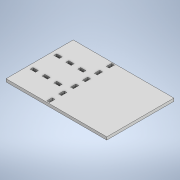
# Autodesk Inventor part: mdf_base_6x6
Saved by Autodesk Inventor 2021.2 (Build 252289000, 289)
## iProperties
Created: 2021-03-24
Part Number: mdf_base_6x6
Material: Generic
Document SubType Name: Modeling
Designer: yxion
Density: 1 g/cm^3
Appearance: Default
Author: yxion
Autodesk Inventor part; units mm, degrees
ref_plane "YZ Plane" through (0, 0, 0) normal (1, 0, 0) x (0, 1, 0)
ref_plane "XZ Plane" through (0, 0, 0) normal (0, 1, 0) x (-1, 0, 0)
ref_plane "XY Plane" through (0, 0, 0) normal (0, 0, 1) x (1, 0, 0)
sketch "Sketch1" plane through (0, 0, 0) normal (0, 1, 0) x (-1, 0, 0)
  line L0 (55.1775, 69.7485) -> (-173.4225, 69.7485)
  line L1 (-173.4225, 69.7485) -> (-173.4225, -82.6515)
  line L2 (-173.4225, -82.6515) -> (55.1775, -82.6515)
  line L3 (55.1775, -82.6515) -> (55.1775, 69.7485)
  point P0 (0, 0)
  dimension "d0" = 152.4
  dimension "d1" = 228.6
  constraints: 8 end point, 2 parallel, 1 horizontal, 1 perpendicular
  measures "d0" distance of L2.end L0.start
  measures "d1" distance of L0.start L0.end
extrude "Extrusion1" add sketch "Sketch1" along normal blind 6.4
sketch "Sketch2" plane through (0, 6.4, 0) normal (0, 1, 0) x (1, 0, 0)
  line L0 (34.6225, 25.9515) -> (41.0225, 25.9515)
  line L1 (41.0225, 25.9515) -> (41.0225, 13.9515)
  line L2 (41.0225, 13.9515) -> (34.6225, 13.9515)
  line L3 (34.6225, 13.9515) -> (34.6225, 25.9515)
  line L4 (34.6225, -1.0485) -> (41.0225, -1.0485)
  line L5 (41.0225, -1.0485) -> (41.0225, -13.0485)
  line L6 (41.0225, -13.0485) -> (34.6225, -13.0485)
  line L7 (34.6225, -13.0485) -> (34.6225, -1.0485)
  line L8 (-55.1775, 82.6515) -> (-55.1775, -69.7485) projected
  line L9 (173.4225, -69.7485) -> (173.4225, 82.6515) construction
  line L10 (173.4225, 82.6515) -> (-55.1775, 82.6515) construction
  line L11 (59.1225, 82.6515) -> (59.1225, -69.7485) construction
  line L12 (-55.1775, -69.7485) -> (173.4225, -69.7485) construction
  line L13 (-55.1775, 6.4515) -> (173.4225, 6.4515) construction
  line L14 (41.0225, -28.0485) -> (41.0225, -40.0485)
  line L15 (34.6225, -40.0485) -> (34.6225, -28.0485)
  line L16 (41.0225, -40.0485) -> (34.6225, -40.0485)
  line L17 (34.6225, -28.0485) -> (41.0225, -28.0485)
  line L18 (41.0225, -55.0485) -> (41.0225, -67.0485)
  line L19 (34.6225, -67.0485) -> (34.6225, -55.0485)
  line L20 (41.0225, -67.0485) -> (34.6225, -67.0485)
  line L21 (34.6225, -55.0485) -> (41.0225, -55.0485)
  line L22 (41.0225, 52.9515) -> (41.0225, 40.9515)
  line L23 (34.6225, 40.9515) -> (34.6225, 52.9515)
  line L24 (34.6225, 52.9515) -> (41.0225, 52.9515)
  line L25 (41.0225, 40.9515) -> (34.6225, 40.9515)
  line L26 (41.0225, 79.9515) -> (41.0225, 67.9515)
  line L27 (34.6225, 67.9515) -> (34.6225, 79.9515)
  line L28 (34.6225, 79.9515) -> (41.0225, 79.9515)
  line L29 (41.0225, 67.9515) -> (34.6225, 67.9515)
  line L30 (7.6225, -17.3485) -> (19.6225, -17.3485)
  line L31 (19.6225, -17.3485) -> (19.6225, -23.7485)
  line L32 (19.6225, -23.7485) -> (7.6225, -23.7485)
  line L33 (7.6225, -23.7485) -> (7.6225, -17.3485)
  line L34 (37.8225, -13.0485) -> (37.8225, -28.0485) construction
  line L35 (7.6225, -20.5485) -> (19.6225, -20.5485) construction
  line L36 (7.6225, 36.6515) -> (19.6225, 36.6515)
  line L37 (19.6225, 36.6515) -> (19.6225, 30.2515)
  line L38 (19.6225, 30.2515) -> (7.6225, 30.2515)
  line L39 (7.6225, 30.2515) -> (7.6225, 36.6515)
  line L40 (19.6225, 33.4515) -> (7.6225, 33.4515) construction
  line L41 (-7.3775, 30.2515) -> (-19.3775, 30.2515)
  line L42 (-19.3775, 30.2515) -> (-19.3775, 36.6515)
  line L43 (-19.3775, 36.6515) -> (-7.3775, 36.6515)
  line L44 (-7.3775, 36.6515) -> (-7.3775, 30.2515)
  line L45 (-19.3775, -17.3485) -> (-7.3775, -17.3485)
  line L46 (-7.3775, -23.7485) -> (-19.3775, -23.7485)
  line L47 (-7.3775, -17.3485) -> (-7.3775, -23.7485)
  line L48 (-19.3775, -23.7485) -> (-19.3775, -17.3485)
  line L49 (-34.3775, 30.2515) -> (-46.3775, 30.2515)
  line L50 (-46.3775, 30.2515) -> (-46.3775, 36.6515)
  line L51 (-46.3775, 36.6515) -> (-34.3775, 36.6515)
  line L52 (-34.3775, 36.6515) -> (-34.3775, 30.2515)
  line L53 (-46.3775, -17.3485) -> (-34.3775, -17.3485)
  line L54 (-34.3775, -23.7485) -> (-46.3775, -23.7485)
  line L55 (-34.3775, -17.3485) -> (-34.3775, -23.7485)
  line L56 (-46.3775, -23.7485) -> (-46.3775, -17.3485)
  point P0 (0, 0)
  point P1 (-19.3775, 33.4515)
  point P2 (-7.3775, 33.4515)
  point P3 (-7.3775, -20.5485)
  point P4 (-19.3775, -20.5485)
  point P5 (-46.3775, 33.4515)
  point P6 (-34.3775, 33.4515)
  point P7 (-34.3775, -20.5485)
  point P8 (-46.3775, -20.5485)
  dimension "d4" = 6.4
  dimension "d5" = 12
  dimension "d6" = 6.4
  dimension "d7" = 12
  dimension "d8" = 15
  dimension "d12" = 7.5
  dimension "d13" = 96.2
  dimension "d14" = 96.2
  dimension "d17" = 27
  dimension "d24" = 27
  dimension "d31" = 6.4
  dimension "d32" = 12
  dimension "d34" = 7.5
  dimension "d35" = 12
  dimension "d36" = 6.4
  dimension "d37" = 7.5
  dimension "d40" = 2.7
  dimension "d41" = 15
  dimension "d42" = 15
  dimension "d45" = 27
  dimension "d50" = 46
  dimension "d51" = 46
  dimension "d52" = 47.6
  dimension "d53" = 89.8
  constraints: 106 end point, 10 midpoint, 8 parallel, 5 horizontal, 4 perpendicular, 3 collinear, 2 vertical, 69 other
  measures "d4" distance of L0.start L0.end
  measures "d5" distance of L0.end L1.end
  measures "d6" distance of L4.start L4.end
  measures "d7" distance of L4.end L5.end
  measures "d8" distance between parallel lines of L4 L2
  measures "d12" distance between parallel lines of L2 L13
  measures "d13" distance between parallel lines of L8 L1
  measures "d14" distance between parallel lines of L8 L5
  measures "d17" distance of L4.end L14.start
  measures "d24" distance of L0.end L22.start
  measures "d31" distance of L30.end L31.end
  measures "d32" distance of L31.end L32.end
  measures "d34" distance between parallel lines of L35 L6
  measures "d35" distance of L36.start L36.end
  measures "d36" distance of L38.end L36.start
  measures "d37" distance between parallel lines of L0 L40
  measures "d40" distance between parallel lines of L12 L20
  measures "d41" distance between parallel lines of L37 L23
  measures "d42" distance from line of L35.end L7
  measures "d45" distance of L37.end L41.start
  measures "d50" distance between parallel lines of L54 L12
  measures "d51" distance between parallel lines of L10 L51
  measures "d52" distance between parallel lines of L53 L49
  measures "d53" distance between parallel lines of L8 L15
extrude "Extrusion2" cut sketch "Sketch2" against normal blind 6.4
equation "\"d29\" = d31"
body "Solid1"
